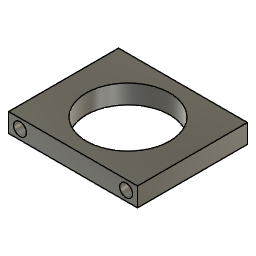
Tube_Joint_Save (Autodesk Fusion 360 archive; units mm, degrees)
design "22mm Tube Clamp"
Autodesk Fusion 360 part; units mm, degrees
sketch "Sketch1" plane through (0, 0, 0) normal (0, 0, 1) x (1, 0, 0)
  line L0 (0, 0) -> (34, 0)
  line L1 (34, 0) -> (34, -29)
  line L2 (34, -29) -> (0, -29)
  line L3 (0, -29) -> (0, 0)
  circle A0 centre (17, -14.5) radius 11
  dimension "d1" = 34
  dimension "d2" = 29
  dimension "d3" = 22
  constraint horizontal L0
  constraint vertical L1
  constraint horizontal L2
  constraint vertical L3
  constraint coincident L0.start L3.end
  measures "d1" distance of L0.start L0.end
  measures "d2" distance of L0.start L2.end
  measures "d3" diameter of A0
extrude "Extrude1" add sketch "Sketch1" along normal blind 5
sketch "Sketch2" plane through (0, 0, 0) normal (0, 1, 0) x (1, 0, 0)
  circle A0 centre (3, -2.5) radius 1.7
  circle A1 centre (31, -2.5) radius 1.7
  dimension "d6" = 3.4
  dimension "d7" = 3.4
  measures "d6" diameter of A0
  measures "d7" diameter of A1
extrude "Extrude2" cut sketch "Sketch2" against normal blind 29
